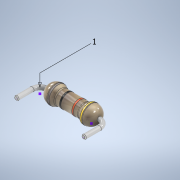
# Autodesk Inventor part: CF14JT10K0
Saved by Autodesk Inventor 2020 (Build 240168000, 168)
## iProperties
Created: 2020-11-14
Part Number: CF14JT10K0
Material: Generic
Document SubType Name: Modeling
Designer: Admin
Density: 1 g/cm^3
Appearance: Default
Author: Admin
Autodesk Inventor part; units mm, degrees
ref_plane "YZ Plane" through (0, 0, 0) normal (1, 0, 0) x (0, 1, 0)
ref_plane "XZ Plane" through (0, 0, 0) normal (0, 1, 0) x (-1, 0, 0)
sketch "Sketch2" plane through (0, 0, 0) normal (0, 0, 1) x (1, 0, 0)
  line L0 (0, 0) -> (0, 0.15)
  line L1 (6.5, 0.15) -> (6.5, 0)
  line L2 (1, 1.15) -> (1.1, 1.15)
  line L3 (5.5, 1.15) -> (5.4, 1.15)
  line L4 (1.6, 1.15) -> (1.6, 1.15)
  line L5 (4.9, 1.15) -> (4.9, 1.15)
  arc A0 (1.7, 0.95) -> (1.85, 0.9) centre (1.85, 1.15) ccw
  arc A1 (4.65, 0.9) -> (4.8, 0.95) centre (4.65, 1.15) ccw
  arc A2 (1.7, 0.95) -> (1.3, 1.1298) centre (1.1, 0.15) ccw
  arc A3 (5.2, 1.1298) -> (4.8, 0.95) centre (5.4, 0.15) ccw
  line L6 (0, 0) -> (1.1, 0)
  arc A4 (6.5, 0.15) -> (5.5, 1.15) centre (5.5, 0.15) ccw
  arc A5 (1, 1.15) -> (0, 0.15) centre (1, 0.15) ccw
  line L7 (1.1, 1.15) -> (1.1, 0)
  line L8 (1.1, 0) -> (1.3, 0)
  line L9 (1.3, 0) -> (1.3, 1.1298)
  line L10 (2.3721, 0.9) -> (2.3721, 0)
  line L11 (2.3721, 0) -> (2.5721, 0)
  line L12 (2.5721, 0) -> (2.5721, 0.9)
  line L13 (2.3721, 0.91) -> (2.5721, 0.91)
  arc A6 (1.3, 1.1398) -> (1.1, 1.16) centre (1.1, 0.16) ccw
  line L14 (5.4, 1.15) -> (5.4, 0)
  line L15 (5.4, 0) -> (5.2, 0)
  line L16 (5.2, 0) -> (5.2, 1.1298)
  line L17 (4.1279, 0.9) -> (4.1279, 0)
  line L18 (4.1279, 0) -> (3.9279, 0)
  line L19 (3.9279, 0) -> (3.9279, 0.9)
  line L20 (4.1279, 0.91) -> (3.9279, 0.91)
  arc A7 (5.4, 1.16) -> (5.2, 1.1398) centre (5.4, 0.16) ccw
  line L21 (1.85, 0.9) -> (2.3721, 0.9)
  line L22 (2.5721, 0.9) -> (3.9279, 0.9)
  line L23 (4.1279, 0.9) -> (4.65, 0.9)
  line L24 (1.1, 0) -> (1.3, 0)
  line L25 (1.3, 0) -> (2.3721, 0)
  line L26 (2.3721, 0) -> (2.5721, 0)
  line L27 (2.5721, 0) -> (3.9279, 0)
  line L28 (3.9279, 0) -> (4.1279, 0)
  line L29 (4.1279, 0) -> (5.2, 0)
  line L30 (5.2, 0) -> (5.4, 0)
  line L31 (5.4, 0) -> (6.5, 0)
  line L32 (1.1, 1.15) -> (1.1, 1.16)
  line L33 (2.3721, 0.9) -> (2.3721, 0.91)
  line L34 (3.9279, 0.9) -> (3.9279, 0.91)
  line L35 (5.2, 1.1298) -> (5.2, 1.1398)
  line L36 (5.4, 1.15) -> (5.4, 1.16)
  line L37 (4.1279, 0.9) -> (4.1279, 0.91)
  line L38 (2.5721, 0.9) -> (2.5721, 0.91)
  line L39 (1.3, 1.1298) -> (1.3, 1.1398)
  point P0 (0, 0)
  point P1 (5.2, 1.1298)
  point P2 (1.3, 1.1298)
  point P3 (1.3, 1.1298)
  constraints: 80 end point, 20 perpendicular, 18 point on circle, 10 tangent, 10 vertical, 8 centre point, 8 point on line, 2 equal radius, 1 collinear, 1 parallel
revolve "Revolution3" add sketch "Sketch2" angle 360 about axis through (0, 0, 0) along (1, 0, 0) contours L0 A5 L2 L7 L6 | L9 A2 A0 L21 L10 L25 | L12 L22 L19 L27 | L17 L23 A1 A3 L16 L29 | L14 L3 A4 L1 L31
revolve "Revolution4" add sketch "Sketch2" angle 360 about axis through (1.1, 0, 0) along (1, 0, 0) contours L7 L32 A6 L39 L9 L8 | L10 L33 L13 L38 L12 L11 | L19 L34 L20 L37 L17 L18 | L16 L35 A7 L36 L14 L15
sketch "Sketch3" plane through (0, 0, 0) normal (-1, 0, 0) x (0, 0, 1)
  circle A0 centre (0, 0) radius 0.15 projected
  line L0 (-0.15, 0) -> (0.15, 0)
  constraints: 2 end point, 2 point on circle
ref_plane "Work Plane1" through (0, 0, -0.15) normal (0, -1, 0) x (0, 0, 1)
sketch "Sketch4" plane through (0, 0, -0.15) normal (0, -1, 0) x (0, 0, 1)
  line L0 (0.15, 0) -> (0.15, 0)
  line L1 (0, -6.5) -> (0.3, -6.5) projected
  line L2 (0.15, -6.5) -> (0.15, -6.5)
  line L3 (1.15, -7.5) -> (3.15, -7.5)
  line L4 (1.15, 1) -> (3.15, 1)
  arc A0 (1.15, 1) -> (0.15, 0) centre (1.15, 0) ccw
  arc A1 (0.15, -6.5) -> (1.15, -7.5) centre (1.15, -6.5) ccw
  dimension "d9" = 1
  constraints: 8 end point, 4 point on circle, 4 tangent, 2 centre point, 2 horizontal, 2 vertical, 1 equal radius, 1 midpoint
  measures "d9" radius of A0
sketch "Sketch5" plane through (6.5, 0, 0) normal (1, 0, 0) x (0, 0, -1)
  circle A0 centre (0, 0) radius 0.275
  constraints: 1 centre point, 1 coincident
sketch "Sketch6" plane through (0, 0, 0) normal (-1, 0, 0) x (0, 0, 1)
  circle A0 centre (0, 0) radius 0.275
  constraints: 1 centre point, 1 coincident
sweep "Sweep1" add profiles "Sketch6" path "Sketch4" path curves L0 A0 L4
sweep "Sweep2" add profiles "Sketch5" path "Sketch4" path curves L2 A1 L3
extrude "Extrusion1" add sketch "Sketch5" against normal blind 6.5
fillet "Fillet1" radius 0.1 7 edges at (6.5, 0, 0.275) (7.225, 0, 1) (7.225, 0, 3) (0, -0.275, 0) (0, 0.275, 0) (-1.275, 0, 1) (-1.275, 0, 3)
body "Solid2"
